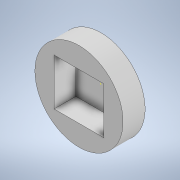
# Autodesk Inventor part: FDMPrintHeadPlanarPrototypes
Saved by Autodesk Inventor 2021 (Build 250183000, 183)
## iProperties
Created: 2022-02-04
Part Number: FDMPrintHeadPlanarPrototypes
Material: Generic
Document SubType Name: Sheet Metal
Designer: Unit-005
Density: 1 g/cm^3
Sheet Metal Rule: Default
Appearance: Default
Author: Unit-005
## iProperties of the stored document _3DPrint.ipt
Created: 2022-02-04
Part Number: _3DPrint
Material: Generic
Document SubType Name: Modeling
Designer: Unit-005
Density: 1 g/cm^3
Appearance: Default
Author: Unit-005
Autodesk Inventor part; units mm, degrees
ref_plane "YZ Plane" through (0, 0, 0) normal (1, 0, 0) x (0, 1, 0)
ref_plane "XZ Plane" through (0, 0, 0) normal (0, 1, 0) x (-1, 0, 0)
ref_plane "XY Plane" through (0, 0, 0) normal (0, 0, 1) x (1, 0, 0)
sketch "Sketch1" plane through (0, 0, 0) normal (0, 0, 1) x (1, 0, 0)
  line L0 (-14.3446, 13.462) -> (14.3446, 13.462)
  line L1 (14.3446, 13.462) -> (14.3446, -13.462)
  line L2 (14.3446, -13.462) -> (-14.3446, -13.462)
  line L3 (-14.3446, -13.462) -> (-14.3446, 13.462)
  line L4 (-14.3446, 13.462) -> (14.3446, -13.462) construction
  line L5 (14.3446, 13.462) -> (-14.3446, -13.462) construction
  point P0 (0, 0)
  dimension "d0" = 28.6893
  dimension "d1" = 26.924
  constraints: 12 end point, 2 midpoint, 2 parallel, 1 horizontal, 1 perpendicular
  measures "d0" distance of L1.end L2.end
  measures "d1" distance of L0.end L1.end
ref_plane "Work Plane1" through (0, 0, 0) normal (0, 0, -1) x (-1, 0, 0)
sketch "Sketch2" plane through (0, 0, 0) normal (0, 0, -1) x (-1, 0, 0)
  circle A0 centre (0, 0) radius 25.4
  dimension "d4" = 50.8
  constraints: 1 centre point, 1 coincident
  measures "d4" diameter of A0
extrude "Extrusion2" add sketch "Sketch2" against normal blind 12.7
extrude "Extrusion3" cut sketch "Sketch1" along normal through all
sketch "Sketch3" plane through (0, 0, 0) normal (0, 0, 1) x (1, 0, 0)
  line L0 (-14.3446, -13.462) -> (14.3446, -13.462) projected
  line L1 (-14.3446, 13.462) -> (-14.3446, -13.462) projected
  line L2 (14.3446, 13.462) -> (-14.3446, 13.462) projected
  line L3 (14.3446, -13.462) -> (14.3446, 13.462) projected
  line L4 (-14.3446, 13.462) -> (-14.3446, -13.462) projected
  line L5 (-14.3446, -13.462) -> (14.3446, -13.462) projected
  line L6 (14.3446, -13.462) -> (14.3446, 13.462) projected
  line L7 (14.3446, 13.462) -> (-14.3446, 13.462) projected
  circle A0 centre (0, 0) radius 25.4 projected
  line L8 (-35.56, 0) -> (35.56, 0) projected
  line L9 (0, -35.56) -> (0, 35.56) projected
  line L10 (14.3446, 13.462) -> (-14.3446, 13.462) projected
  line L11 (-14.3446, -13.462) -> (14.3446, -13.462)
  line L12 (14.3446, -13.462) -> (14.3446, 13.462)
  line L13 (14.3446, 13.462) -> (-14.3446, 13.462)
  line L14 (-14.3446, 13.462) -> (-14.3446, -13.462)
  line L15 (-14.3446, -13.462) -> (14.3446, 13.462) construction
  line L16 (14.3446, -13.462) -> (-14.3446, 13.462) construction
  line L17 (14.3446, 13.462) -> (-14.3446, 13.462) projected
  line L18 (-14.3446, -13.462) -> (14.3447, -13.462)
  line L19 (14.3447, -13.462) -> (14.3446, 13.462)
  line L20 (14.3446, 13.462) -> (-14.3446, 13.462)
  line L21 (-14.3446, 13.462) -> (-14.3446, -13.462)
  line L22 (-14.3446, -13.462) -> (14.3446, 13.462) construction
  line L23 (14.3447, -13.462) -> (-14.3446, 13.462) construction
  line L24 (14.3446, -13.462) -> (14.3446, 13.462) projected
  constraints: 24 end point, 5 midpoint, 4 parallel, 3 collinear, 2 horizontal, 2 perpendicular, 1 point on line
extrude "Extrusion4" add sketch "Sketch3" along normal blind 0.1524 contours L1 L8 L9 L0 | L9 L8 L3 L0 | L1 L2 L9 L8 | L9 L2 L3 L8
pattern_linear "Rectangular Pattern1" [suppressed]
sketch "Sketch4" plane through (0, 0, 0) normal (0, 0, 1) x (1, 0, 0)
  circle A0 centre (0, 0) radius 25.4 projected
  line L0 (-35.56, 0) -> (35.56, 0) projected
  line L1 (0, -35.56) -> (0, 35.56) projected
  line L2 (-14.3446, -13.462) -> (14.3446, -13.462) projected
  line L3 (13.5954, 13.462) -> (13.5954, -13.462) projected
  line L4 (-12.1856, -13.462) -> (13.5954, -13.462)
  line L5 (13.5954, -13.462) -> (13.5954, -0.254)
  line L6 (13.5954, -0.254) -> (-12.1857, -0.254)
  line L7 (-12.1857, -0.254) -> (-12.1856, -13.462)
  line L8 (13.2144, 13.462) -> (13.5954, 13.462)
  line L9 (10.6744, 13.462) -> (11.0554, 13.462)
  line L10 (8.1344, 13.462) -> (8.5154, 13.462)
  line L11 (5.5944, 13.462) -> (5.9754, 13.462)
  line L12 (3.0544, 13.462) -> (3.4354, 13.462)
  line L13 (0.5144, 13.462) -> (0.8954, 13.462)
  line L14 (-2.0256, 13.462) -> (-1.6446, 13.462)
  line L15 (-4.5656, 13.462) -> (-4.1846, 13.462)
  line L16 (-7.1056, 13.462) -> (-6.7246, 13.462)
  line L17 (-9.6456, 13.462) -> (-9.2646, 13.462)
  line L18 (-12.1856, 13.462) -> (-11.8046, 13.462)
  line L19 (-12.1856, 13.462) -> (-11.8046, 13.462)
  line L20 (-12.1856, 13.462) -> (13.5954, 13.462)
  line L21 (13.5954, 13.462) -> (13.5954, 0.254)
  line L22 (13.5954, 0.254) -> (-12.1857, 0.254)
  line L23 (-12.1857, 0.254) -> (-12.1856, 13.462)
  point P0 (-11.8046, -13.462)
  dimension "d15" = 0.254
  constraints: 40 end point, 4 symmetric about line, 2 parallel, 1 horizontal, 1 perpendicular, 1 point on line
  measures "d15" distance between parallel lines of L0 L6
extrude "Extrusion5" [suppressed]
sketch "Sketch5" plane through (0, 0, 0) normal (0, 0, -1) x (-1, 0, 0)
  circle A0 centre (0, 0) radius 25.4 projected
  line L0 (35.56, 0) -> (-35.56, 0) projected
  line L1 (0, -35.56) -> (0, 35.56) projected
  circle A1 centre (11.9952, -2.794) radius 0.5
  point P0 (11.9952, -0.254)
  dimension "d18" = 1
  constraints: 1 centre point, 1 vertical alignment
  measures "d18" diameter of A1
extrude "Extrusion6" [suppressed]
pattern_linear "Rectangular Pattern2" [suppressed]
mirror "Mirror1" [suppressed]
sketch "Sketch6" plane through (0, 0, 0) normal (0, 0, -1) x (-1, 0, 0)
  point P0 (0, 0)
equation "\"BendRadius\" = Thickness"
equation "\"BendReliefWidth\" = Thickness"
equation "\"BendReliefDepth\" = 0.5 * Thickness"
equation "\"CornerReliefSize\" = 4 * Thickness"
equation "\"MinimumRemnant\" = 2 * Thickness"
equation "\"TransitionRadius\" = BendRadius"
equation "\"JacobiRadiusSize\" = BendRadius"
equation "\"GapSize\" = Thickness"
equation "\"Thickness\" = 3.048"
body "Solid2"
